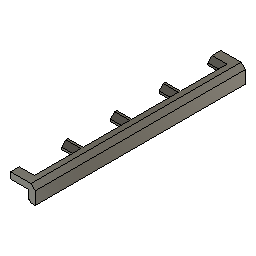
Haltebügel_Ampelsteuerung (Autodesk Fusion 360 design; units mm, degrees)
Autodesk Fusion 360 part; units mm, degrees
sketch "Skizze1" plane through (0, 0, 14) normal (0, 0, 1) x (-1, 0, 0) in component "Haltebügel_Steckverbinder"
  line L0 (105, -43.5) -> (105, -57)
  line L1 (105, -57) -> (105.5, -57)
  line L2 (105.5, -57) -> (105.5, -50)
  line L3 (105.5, -50) -> (112.5, -50)
  line L4 (112.5, -50) -> (112.5, -43.5)
  line L5 (112.5, -43.5) -> (105, -43.5)
  line L6 (112.5, -50) -> (105, -50)
  line L7 (105, -50) -> (105, 43.5)
  line L8 (105, 43.5) -> (112.5, 43.5)
  line L9 (112.5, 43.5) -> (112.5, -50)
  line L10 (105, -43.5) -> (108.5, -43.5)
  line L11 (108.5, -43.5) -> (108.5, -25.5)
  line L12 (108.5, -25.5) -> (105, -25.5)
  line L13 (105, -25.5) -> (105, -43.5)
  line L14 (105, -20.5) -> (108.5, -20.5)
  line L15 (108.5, -20.5) -> (108.5, -2.5)
  line L16 (108.5, -2.5) -> (105, -2.5)
  line L17 (105, -2.5) -> (105, -20.5)
  line L18 (105, 2.5) -> (108.5, 2.5)
  line L19 (108.5, 2.5) -> (108.5, 20.5)
  line L20 (108.5, 20.5) -> (105, 20.5)
  line L21 (105, 20.5) -> (105, 2.5)
  line L22 (105, 25.5) -> (108.5, 25.5)
  line L23 (108.5, 25.5) -> (108.5, 43.5)
  line L24 (108.5, 43.5) -> (105, 43.5)
  line L25 (105, 43.5) -> (105, 25.5)
  line L26 (105, 43.5) -> (112.5, 43.5)
  line L27 (112.5, 43.5) -> (112.5, 50)
  line L28 (112.5, 50) -> (105, 50)
  line L29 (105, 50) -> (105, 43.5)
  line L30 (108.5, 25.5) -> (112.5, 25.5)
  line L31 (108.5, 20.5) -> (112.5, 20.5)
  line L32 (108.5, 2.5) -> (112.5, 2.5)
  line L33 (108.5, -2.5) -> (112.5, -2.5)
  line L34 (108.5, -20.5) -> (112.5, -20.5)
  line L35 (108.5, -25.5) -> (112.5, -25.5)
  line L36 (108.5, -43.5) -> (112.5, -43.5)
  dimension "d187_1" = 3.5
  dimension "d188_1" = 3.5
  dimension "d189_1" = 18
  dimension "d190_1" = 3.5
  dimension "d191_1" = 18
  dimension "d192_1" = 3.5
  dimension "d193_1" = 18
  constraint horizontal L6
  constraint vertical L7
  constraint horizontal L8
  constraint vertical L9
  constraint coincident L3.end L4.start
  constraint horizontal L10
  constraint vertical L11
  constraint horizontal L12
  constraint vertical L13
  constraint coincident L0.start L5.end
  constraint horizontal L14
  constraint vertical L15
  constraint horizontal L16
  constraint vertical L17
  constraint coincident L7 L14.start
  constraint horizontal L18
  constraint vertical L19
  constraint horizontal L20
  constraint vertical L21
  constraint coincident L7 L18.start
  constraint horizontal L22
  constraint vertical L23
  constraint horizontal L24
  constraint vertical L25
  constraint coincident L7 L22.start
  constraint horizontal L26
  constraint vertical L27
  constraint horizontal L28
  constraint vertical L29
  constraint coincident L9 L30.end
  constraint perpendicular L9 L30
  constraint coincident L9 L31.end
  constraint perpendicular L9 L31
  constraint coincident L9 L32.end
  constraint perpendicular L9 L32
  constraint coincident L9 L33.end
  constraint perpendicular L9 L33
  constraint coincident L9 L34.end
  constraint perpendicular L9 L34
  constraint coincident L9 L35.end
  constraint perpendicular L9 L35
  constraint coincident L4.end L5.start
  measures "d187_1" distance of L0.start L10.end
  measures "d188_1" distance of L14.start L14.end
  measures "d189_1" distance of L14.start L16.end
  measures "d190_1" distance of L18.start L18.end
  measures "d191_1" distance of L18.start L20.end
  measures "d192_1" distance of L22.start L22.end
  measures "d193_1" distance of L22.start L7.end
extrude "Extrusion1" add sketch "Skizze1" along normal blind 3 contours L0 L3 L4 L5 L6 L7 L9 L10 L36 | L5 L7 L10 L11 L12 L13 | L7 L9 L12 L14 L34 L35 | L7 L14 L15 L16 L17 | L7 L9 L16 L18 L32 L33 | L7 L18 L19 L20 L21 | L7 L9 L20 L22 L30 L31 | L7 L8 L22 L23 L24 L25 L26 | L8 L24 L26 L27 L28 L29 in component "Haltebügel_Steckverbinder"
extrude "Extrusion2" add 9 faces at (-105, -47.8333, 15) (-105, -31.5, 15) (-105, -22.1667, 15) (-105, -8.5, 15) (-105, 0.8333, 15) (-105, 14.5, 15) (-105, 23.8333, 15) (-105, 37.5, 15) (-105, 45.6667, 15) along direction (1, 0, 0) blind 1.5 in component "Haltebügel_Steckverbinder"
sketch "Skizze2" plane through (-103.5, 0, 0) normal (1, 0, 0) x (0, 1, 0) in component "Haltebügel_Steckverbinder"
  line L0 (-50, 14) -> (50, 14)
  line L1 (50, 14) -> (50, 17)
  line L2 (50, 17) -> (-50, 17)
  line L3 (-50, 17) -> (-50, 14)
  line L4 (-50, 17) -> (50, 17)
  line L5 (50, 17) -> (50, 9)
  line L6 (50, 9) -> (-50, 9)
  line L7 (-50, 9) -> (-50, 17)
  dimension "d198_1" = 8
  constraint horizontal L4
  constraint vertical L5
  constraint horizontal L6
  constraint vertical L7
  constraint coincident L2.end L3.start
  measures "d198_1" distance of L2.end L6.end
extrude "Extrusion3" add sketch "Skizze2" along normal blind 3 in component "Haltebügel_Steckverbinder"
extrude "Extrusion4" cut 4 faces at (-108.5, 37.5, 15) (-108.5, 14.5, 15) (-108.5, -8.5, 16) (-108.5, -31.5, 15) along direction (1, 0, 0) blind 1.5 in component "Haltebügel_Steckverbinder"
extrude "Extrusion5" cut 1 faces at (-105.5, 50, 16) along direction (0, -1, 0) blind 0.4 in component "Haltebügel_Steckverbinder"
extrude "Extrusion6" cut 1 faces at (-105.5, -50, 16) along direction (0, 1, 0) blind 0.4 in component "Haltebügel_Steckverbinder"
chamfer "Fase1" distance 2 angle 45 1 edges at (-100.5, 0, 17) in component "Haltebügel_Steckverbinder"
chamfer "Fase2" distance 1 angle 45 1 edges at (-103.5, 0, 9) in component "Haltebügel_Steckverbinder"
chamfer "Fase3" distance 2 angle 45 12 edges at (-107, 34.5, 17) (-107, 11.5, 17) (-107, -11.5, 17) (-107, -34.5, 17) (-109.75, -43.5, 17) (-109.75, -25.5, 17) (-109.75, -20.5, 17) (-109.75, -2.5, 17) (-109.75, 2.5, 17) (-109.75, 20.5, 17) (-109.75, 25.5, 17) (-109.75, 43.5, 17) in component "Haltebügel_Steckverbinder"
extrude "Extrusion7" cut 5 faces at (-112.5, 46.2, 15) (-112.5, 22.8333, 15.6667) (-112.5, 0.1667, 15) (-112.5, -22.8333, 15) (-112.5, -46.2, 15) along direction (1, 0, 0) blind 0.4 in component "Haltebügel_Steckverbinder"
component "Haltebügel_Steckverbinder" placed x (1, 0, 0) y (0, 1, 0) z (0, 0, 1) at (0, 0, 0)
